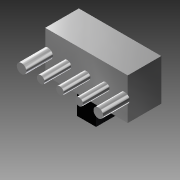
# Autodesk Inventor part: TE-1825232
Saved by Autodesk Inventor 2016 (Build 200138000, 138)
## iProperties
Created: 2017-02-23
Part Number: TE-1825232
Material: Generic
Document SubType Name: Modeling
Designer: Tyler
Density: 1 g/cm^3
Appearance: Chrome - Polished
Author: Tyler
Autodesk Inventor part; units mm, degrees
ref_plane "YZ Plane" through (0, 0, 0) normal (1, 0, 0) x (0, 1, 0)
ref_plane "XZ Plane" through (0, 0, 0) normal (0, 1, 0) x (-1, 0, 0)
sketch "Sketch1" plane through (0, 0, 0) normal (0, 1, 0) x (-1, 0, 0)
  line L0 (-4.3, 2.15) -> (4.3, 2.15)
  line L1 (4.3, 2.15) -> (4.3, -2.15)
  line L2 (4.3, -2.15) -> (-4.3, -2.15)
  line L3 (-4.3, -2.15) -> (-4.3, 2.15)
  line L4 (-4.3, 2.15) -> (4.3, -2.15) construction
  line L5 (4.3, 2.15) -> (-4.3, -2.15) construction
  point P0 (0, 0)
  dimension "d0" = 8.6
  dimension "d1" = 4.3
  constraints: 12 end point, 2 midpoint, 2 parallel, 1 horizontal, 1 perpendicular
  measures "d0" distance of L1.end L2.end
  measures "d1" distance of L0.end L1.end
extrude "Extrusion1" add sketch "Sketch1" along normal blind 3.5
sketch "Sketch2" plane through (0, 0, 0) normal (0, -1, 0) x (1, 0, 0)
  circle A0 centre (0, 0) radius 0.4
  circle A1 centre (2, 0) radius 0.4
  circle A2 centre (-2, 0) radius 0.4
  circle A3 centre (-4, 0) radius 0.5
  circle A4 centre (4, 0) radius 0.5
  dimension "d4" = 0.8
  dimension "d5" = 0.8
  dimension "d6" = 0.8
  dimension "d7" = 2
  dimension "d8" = 2
  dimension "d9" = 1
  dimension "d10" = 1
  dimension "d11" = 2
  dimension "d12" = 2
  constraints: 5 centre point, 1 coincident
  measures "d4" diameter of A0
  measures "d5" diameter of A1
  measures "d6" diameter of A2
  measures "d7" distance of A0.centre A2.centre
  measures "d8" distance of point (0, 0) A1.centre
  measures "d9" diameter of A3
  measures "d10" diameter of A4
  measures "d11" distance of A2.centre A3.centre
  measures "d12" distance of A1.centre A4.centre
extrude "Extrusion2" add sketch "Sketch2" along normal blind 2.77
ref_plane "Work Plane1" through (0, 2, 0) normal (0, -1, 0) x (1, 0, 0)
sketch "Sketch3" plane through (0, 2, 0) normal (0, -1, 0) x (1, 0, 0)
  line L0 (-2, -2.15) -> (-2, -5.15)
  line L1 (-2, -5.15) -> (0, -5.15)
  line L2 (-2, -2.15) -> (0, -2.15)
  line L3 (0, -2.15) -> (0, -5.15)
  line L4 (-4.3, -2.15) -> (4.3, -2.15) projected
  point P0 (0, 0)
  dimension "d16" = 2
  dimension "d17" = 0
  dimension "d18" = 0
  dimension "d19" = 3
  constraints: 8 end point, 2 perpendicular, 1 parallel, 1 vertical
  measures "d16" distance of L0.start L2.end
  measures "d17" distance from line of point (0, 0) L3
  measures "d18" distance between parallel lines of L4 L2
  measures "d19" distance of L0.start L0.end
extrude "Extrusion3" add sketch "Sketch3" along normal mid plane 2
body "Solid1"
